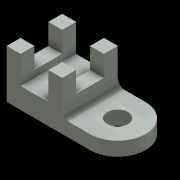
# Autodesk Inventor part: tut
Saved by Autodesk Inventor 2015 SP2 (Build 190223200, 223)
## iProperties
Created: 2015-09-23
Part Number: tut
Material: Titanium
Document SubType Name: Modeling
Designer: Brandon
Mass: 431.707 g
Surface Area: 202.059 cm^2
Volume: 95.7223 cm^3
Density: 4.51 g/cm^3
Appearance: Titanium
Author: Brandon
Autodesk Inventor part; units mm, degrees
ref_plane "YZ Plane" through (0, 0, 0) normal (1, 0, 0) x (0, 1, 0)
ref_plane "XZ Plane" through (0, 0, 0) normal (0, 1, 0) x (-1, 0, 0)
ref_plane "XY Plane" through (0, 0, 0) normal (0, 0, 1) x (1, 0, 0)
sketch "Sketch1" plane through (0, 0, 0) normal (0, 0, 1) x (1, 0, 0)
  line L0 (0, 0) -> (76.2, 0)
  line L1 (76.2, 0) -> (76.2, 12.7)
  line L2 (0, 0) -> (0, 44.45)
  line L3 (0, 44.45) -> (12.7, 44.45)
  line L4 (12.7, 44.45) -> (12.7, 19.05)
  line L5 (12.7, 19.05) -> (38.1, 19.05)
  line L6 (38.1, 19.05) -> (38.1, 44.45)
  line L7 (38.1, 44.45) -> (50.8, 44.45)
  line L8 (50.8, 44.45) -> (50.8, 19.05)
  line L9 (57.15, 12.7) -> (76.2, 12.7)
  arc A0 (50.8, 19.05) -> (57.15, 12.7) centre (57.15, 19.05) ccw
  point P0 (50.8, 12.7)
  dimension "d1" = 12.7
  dimension "d2" = 44.45
  dimension "d3" = 12.7
  dimension "d6" = 12.7
  dimension "d7" = 76.2
  dimension "d8" = 50.8
  dimension "d9" = 19.05
  dimension "d28" = 6.35
  constraints: 20 end point, 6 perpendicular, 4 point on line, 2 point on circle, 2 tangent, 2 vertical, 1 centre point, 1 horizontal
  measures "d1" distance of L0.end L1.end
  measures "d2" distance of L0.start L2.end
  measures "d3" distance of L2.end L3.end
  measures "d6" distance of L6.end L7.end
  measures "d7" distance of L0.start L0.end
  measures "d8" distance of L7.end L2.end
  measures "d9" distance between parallel lines of L0 L5
  measures "d28" radius of A0
extrude "Base" add sketch "Sketch1" along normal blind 50.8
sketch "Sketch2" plane through (50.8, 12.7, 0) normal (0, 1, 0) x (1, 0, 0)
  line L0 (25.4, 0) -> (25.4, -50.8) projected
  circle A0 centre (25.4, -25.4) radius 25.4
  point P0 (-50.8, 0)
  constraints: 1 midpoint, 1 vertical alignment, 2 other
extrude "Ciclre" add sketch "Sketch2" against normal blind 12.7
hole "Hole1" at (76.2, 0, 25.4) direction (0, 1, 0) diameter 19.05 end through all
sketch "Sketch4" plane through (50.8, 12.7, 0) normal (1, 0, 0) x (0, 0, -1)
  line L0 (-50.8, 31.75) -> (-38.1, 31.75)
  line L1 (0, 31.75) -> (-50.8, 31.75) projected
  line L2 (-38.1, 31.75) -> (-38.1, 12.7)
  line L3 (-38.1, 12.7) -> (-12.7, 12.7)
  line L4 (-12.7, 12.7) -> (-12.7, 31.75)
  line L5 (-38.1, 31.75) -> (-12.7, 31.75)
  line L6 (0, 31.75) -> (-50.8, 31.75) projected
  point P0 (0, -12.7)
  dimension "d23" = 12.7
  dimension "d24" = 19.05
  dimension "d25" = 25.4
  constraints: 10 end point, 2 perpendicular, 2 point on line, 1 collinear, 1 vertical
  measures "d23" distance of L0.start L0.end
  measures "d24" distance of L0.end L2.end
  measures "d25" distance of L2.end L3.end
extrude "Extrusion3" cut sketch "Sketch4" against normal through all
body "Solid1"
